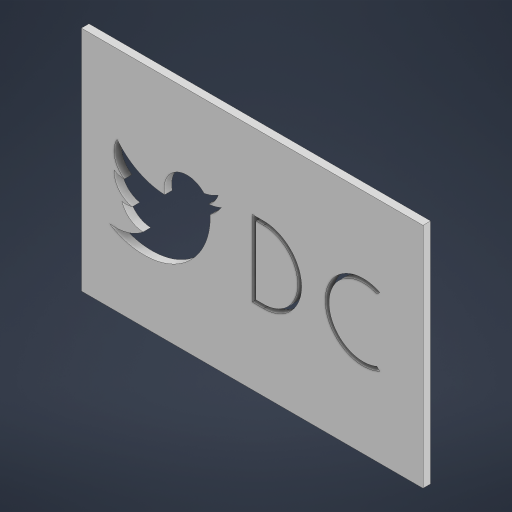
# Autodesk Inventor part: Workspacev3
Saved by Autodesk Inventor 2023.4 (Build 274418000, 418)
## iProperties
Created: 2024-02-24
Part Number: Workspacev3
Material: Generic
Document SubType Name: Modeling
Designer: ASUS
Density: 1 g/cm^3
Appearance: Default
Author: ASUS
Autodesk Inventor part; units mm, degrees
ref_plane "YZ Plane" through (0, 0, 0) normal (1, 0, 0) x (0, 1, 0)
ref_plane "XZ Plane" through (0, 0, 0) normal (0, 1, 0) x (-1, 0, 0)
ref_plane "XY Plane" through (0, 0, 0) normal (0, 0, 1) x (1, 0, 0)
sketch "Sketch3" plane through (0, 0, 0) normal (0, 0, 1) x (1, 0, 0)
  line L0 (225, -150) -> (-225, -150)
  line L1 (-225, -150) -> (-225, 150)
  line L2 (-225, 150) -> (225, 150)
  line L3 (225, 150) -> (225, -150)
  line L4 (225, -150) -> (-225, 150) construction
  line L5 (-225, -150) -> (225, 150) construction
  point P0 (0, 0)
  dimension "d28" = 450
  dimension "d29" = 300
  constraints: 12 end point, 2 midpoint, 2 parallel, 1 horizontal, 1 perpendicular
  measures "d28" distance of L1.end L2.end
  measures "d29" distance of L0.end L1.end
extrude "Extrusion3" add sketch "Sketch3" against normal blind 10
sketch "Sketch4" plane through (0, 0, 0) normal (0, 0, 1) x (1, 0, 0)
  line L0 (-188.5773, 52.7966) -> (-39.7688, 52.7966) construction
  line L1 (-39.7688, 52.7966) -> (-39.7688, -69.5636) construction
  line L2 (-39.7688, -69.5636) -> (-188.5773, -69.5636) construction
  line L3 (-188.5773, -69.5636) -> (-188.5773, 52.7966) construction
  arc A0 (-63.474, 42.3636) -> (-115.2717, 14.7448) centre (-85.6644, 21.5993) ccw
  arc A1 (-63.474, 42.3636) -> (-44.7993, 49.5387) centre (-72.9613, 94.9469) ccw
  arc A2 (-57.5211, 33.0678) -> (-44.7993, 49.5387) centre (-73.5639, 58.6073) ccw
  arc A3 (-57.5211, 33.0678) -> (-40.4668, 37.5486) centre (-61.5692, 83.1704) ccw
  arc A4 (-55.279, 22.1457) -> (-40.4668, 37.5486) centre (-91.7711, 72.0616) ccw
  arc A5 (-187.84, -54.5358) -> (-55.279, 22.1457) centre (-142.1639, 19.4243) ccw
  arc A6 (-187.84, -54.5358) -> (-143.6311, -41.8595) centre (-180.716, 4.0471) ccw
  arc A7 (-171.5212, -21.0902) -> (-143.6311, -41.8595) centre (-142.8553, -11.7068) ccw
  arc A8 (-171.5212, -21.0902) -> (-157.9673, -20.3144) centre (-166.5282, 10.4646) ccw
  arc A9 (-181.9106, 9.4083) -> (-157.9673, -20.3144) centre (-152.8099, 8.3454) ccw
  arc A10 (-181.9106, 9.4083) -> (-168.3407, 6.1387) centre (-169.5368, 30.9698) ccw
  arc A11 (-177.8021, 46.6432) -> (-168.3407, 6.1387) centre (-151.8985, 31.3367) ccw
  arc A12 (-177.8021, 46.6432) -> (-115.2717, 14.7448) centre (-111.5306, 99.3167) ccw
  line L4 (0, 50) -> (0, -50)
  line L5 (0, 50) -> (15, 50)
  line L6 (0, -50) -> (15, -50)
  arc A13 (15, -50) -> (15, 50) centre (15, 0) ccw
  line L7 (15, 45) -> (5, 45)
  line L8 (5, 45) -> (5, -45)
  line L9 (5, -45) -> (15, -45)
  arc A14 (15, -45) -> (15, 45) centre (15, 0) ccw
  arc A15 (174.4806, 41.2317) -> (167.9918, 45) centre (146.1973, 0) ccw construction
  arc A16 (164.2235, -41.2317) -> (164.2235, 41.2317) centre (146.1973, 0) ccw construction
  line L10 (167.9918, 45) -> (167.9918, -45) construction
  line L11 (167.9918, 45) -> (164.2235, 41.2317)
  line L12 (164.2235, 41.2317) -> (184.5876, 41.2317) construction
  line L13 (164.2235, 41.2317) -> (164.2235, -41.2317) construction
  line L14 (167.9918, -45) -> (164.2235, -41.2317)
  arc A17 (164.2235, 41.2317) -> (164.2235, -41.2317) centre (146.1973, 0) ccw
  arc A18 (167.9918, -45) -> (174.4806, 41.2317) centre (146.1973, 0) ccw construction
  line L15 (164.2235, -41.2317) -> (164.2235, -55.8209) construction
  arc A19 (167.9918, 45) -> (167.9918, -45) centre (146.1973, 0) ccw
  point P0 (0, 0)
  dimension "d33" = 100
  dimension "d36" = 50
  dimension "d37" = 15
  dimension "d38" = 15
  dimension "d39" = 5
  dimension "d41" = 5
  dimension "d42" = 45
  constraints: 42 point on circle, 24 end point, 20 centre point, 3 horizontal, 3 vertical, 2 point on line, 1 perpendicular, 1 tangent, 5 other
  measures "d33" distance of L4.start L4.end
  measures "d36" distance of L4.start point (0, 0)
  measures "d37" distance of L4.start L5.end
  measures "d38" distance of L4.end L6.end
  measures "d39" radial gap between concentric circles of A13 A14
  measures "d41" radial gap between concentric circles of A15 A16
  measures "d42" angle of L11 L12
extrude "Extrusion4" cut sketch "Sketch4" against normal through all
equation "\"d36\" = 0.5 * d33"
equation "\"d37\" = d38"
body "Solid2"
